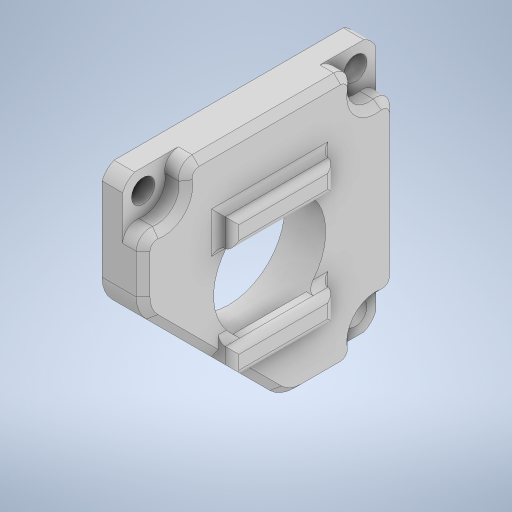
# Autodesk Inventor part: X-Axis-Motor-Support v0.1
Saved by Autodesk Inventor 2023 (Build 270158000, 158)
## iProperties
Created: 2023-07-26
Part Number: X-Axis-Motor-Support v0.1
Material: Generic
Document SubType Name: Modeling
Designer: Parker
Density: 1 g/cm^3
Appearance: Default
Author: Parker
Autodesk Inventor part; units mm, degrees
ref_plane "YZ Plane" through (0, 0, 0) normal (1, 0, 0) x (0, 1, 0)
ref_plane "XZ Plane" through (0, 0, 0) normal (0, 1, 0) x (-1, 0, 0)
ref_plane "XY Plane" through (0, 0, 0) normal (0, 0, 1) x (1, 0, 0)
sketch "Sketch1" plane through (0, 0, 0) normal (1, 0, 0) x (0, 1, 0)
  circle A0 centre (0, 0) radius 8 construction
  circle A1 centre (0, 0) radius 8.2
  line L0 (-15.5, 15.5) -> (15.5, 15.5) construction
  line L1 (15.5, 15.5) -> (15.5, -15.5) construction
  line L2 (15.5, -15.5) -> (-15.5, -15.5) construction
  line L3 (-15.5, -15.5) -> (-15.5, 15.5) construction
  line L4 (-15.5, 15.5) -> (15.5, -15.5) construction
  line L5 (15.5, 15.5) -> (-15.5, -15.5) construction
  line L6 (-18.5, 18.5) -> (18.5, 18.5)
  line L7 (18.5, 18.5) -> (18.5, -18.5)
  line L8 (18.5, -18.5) -> (-18.5, -18.5)
  line L9 (-18.5, -18.5) -> (-18.5, 18.5)
  line L10 (-18.5, 18.5) -> (18.5, -18.5) construction
  line L11 (18.5, 18.5) -> (-18.5, -18.5) construction
  line L12 (-18.5, -2.5) -> (2.5, 18.5)
  point P0 (-15.5, -15.5)
  dimension "d0" = 16
  dimension "d1" = 0.2
  dimension "d2" = 31
  dimension "d3" = 31
  dimension "d4" = 3
  dimension "d5" = 3
  dimension "d6" = 16
  constraints: 26 end point, 5 coincident, 5 parallel, 4 midpoint, 2 centre point, 2 horizontal, 2 perpendicular, 2 point on line
  measures "d0" diameter of A0
  measures "d1" radial gap between concentric circles of A0 A1
  measures "d2" distance of L0.end L1.end
  measures "d3" distance of L0.start L0.end
  measures "d4" distance from line of L8 L1.end
  measures "d5" distance between parallel lines of L7 L1
  measures "d6" distance of L6.end L12.end
extrude "Extrusion1" add sketch "Sketch1" along normal blind 6 contours L6 L7 L8 L9 L12
sketch "Sketch2" plane through (6, 0, 0) normal (1, 0, 0) x (0, 0, -1)
  point P0 (0, 0)
  point P1 (-15.5, 15.5)
  point P2 (15.5, 15.5)
  point P3 (15.5, -15.5)
hole "Hole1" at (6, 15.5, 15.5) at (6, 15.5, -15.5) at (6, -15.5, -15.5) direction (-1, 0, 0) diameter 3.4 end through all counterbore diameter 6.5 counterbore depth 3 clearance for "Socket Head Cap Screw" size "M3" standard "Ansi Metric M Profile"
sketch "Sketch3" plane through (6, 0, 0) normal (1, 0, 0) x (0, 0, -1)
  arc A0 (-16.75, 18.5) -> (-18.5, 16.75) centre (-15.5, 15.5) ccw projected
  line L0 (-16.75, 18.5) -> (-18.5, 18.5) projected
  line L1 (-18.5, 18.5) -> (-18.5, 16.75) projected
  arc A1 (18.5, 16.75) -> (16.75, 18.5) centre (15.5, 15.5) ccw projected
  line L2 (18.5, 16.75) -> (18.5, 18.5) projected
  line L3 (18.5, 18.5) -> (16.75, 18.5) projected
  arc A2 (16.75, -18.5) -> (18.5, -16.75) centre (15.5, -15.5) ccw projected
  line L4 (16.75, -18.5) -> (18.5, -18.5) projected
  line L5 (18.5, -18.5) -> (18.5, -16.75) projected
  point P0 (0, 0)
extrude "Extrusion2" cut sketch "Sketch3" against normal through all
fillet "Fillet1" radius 2 6 edges at (4.5, 14.25, 18.5) (4.5, 18.5, 14.25) (4.5, 18.5, -14.25) (4.5, 14.25, -18.5) (4.5, -14.25, -18.5) (4.5, -18.5, -14.25)
fillet "Fillet2" radius 5 2 edges at (3, 2.5, 18.5) (3, -18.5, -2.5)
sketch "Sketch4" plane through (6, 0, 0) normal (1, 0, 0) x (0, 0, -1)
  circle A0 centre (0, 0) radius 8.2 projected
  arc A1 (1.0355, -17.0355) -> (4.5711, -18.5) centre (4.5711, -13.5) ccw projected
  line L0 (4.5711, -18.5) -> (10.3461, -18.5) projected
  arc A2 (10.3461, -18.5) -> (12.3095, -16.119) centre (10.3461, -16.5) ccw projected
  arc A3 (16.119, -12.3095) -> (12.3095, -16.119) centre (15.5, -15.5) ccw projected
  arc A4 (16.119, -12.3095) -> (18.5, -10.3461) centre (16.5, -10.3461) ccw projected
  line L1 (18.5, -10.3461) -> (18.5, 10.3461) projected
  arc A5 (18.5, 10.3461) -> (16.119, 12.3095) centre (16.5, 10.3461) ccw projected
  arc A6 (12.3095, 16.119) -> (16.119, 12.3095) centre (15.5, 15.5) ccw projected
  arc A7 (12.3095, 16.119) -> (10.3461, 18.5) centre (10.3461, 16.5) ccw projected
  line L2 (10.3461, 18.5) -> (-10.3461, 18.5) projected
  arc A8 (-10.3461, 18.5) -> (-12.3095, 16.119) centre (-10.3461, 16.5) ccw projected
  arc A9 (-16.119, 12.3095) -> (-12.3095, 16.119) centre (-15.5, 15.5) ccw projected
  arc A10 (-16.119, 12.3095) -> (-18.5, 10.3461) centre (-16.5, 10.3461) ccw projected
  line L3 (-18.5, 10.3461) -> (-18.5, 4.5711) projected
  arc A11 (-18.5, 4.5711) -> (-17.0355, 1.0355) centre (-13.5, 4.5711) ccw projected
  line L4 (-17.0355, 1.0355) -> (1.0355, -17.0355) projected
  line L5 (-7.5, 10.2) -> (7.5, 10.2)
  line L6 (7.5, 10.2) -> (7.5, 6.2)
  line L7 (7.5, 6.2) -> (-7.5, 6.2)
  line L8 (-7.5, 6.2) -> (-7.5, 10.2)
  circle A12 centre (0, 0) radius 8.2 projected
  line L9 (-7.5, 10.2) -> (7.5, 6.2) construction
  line L10 (7.5, 10.2) -> (-7.5, 6.2) construction
  line L11 (-7.5, -6.2) -> (7.5, -6.2)
  line L12 (7.5, -6.2) -> (7.5, -10.2)
  line L13 (7.5, -10.2) -> (-7.5, -10.2)
  line L14 (-7.5, -10.2) -> (-7.5, -6.2)
  line L15 (-7.5, -6.2) -> (7.5, -10.2) construction
  line L16 (7.5, -6.2) -> (-7.5, -10.2) construction
  point P0 (0, 8.2)
  point P1 (0, -8.2)
  point P2 (-7.5, -8.5)
  point P3 (-5.8, -10.2)
  dimension "d20" = 15
  dimension "d21" = 4
  dimension "d22" = 15
  dimension "d23" = 4
  constraints: 24 end point, 4 midpoint, 4 parallel, 2 horizontal, 2 perpendicular, 2 point on circle
  measures "d20" distance of L6.end L7.end
  measures "d21" distance of L5.end L6.end
  measures "d22" distance of L12.end L13.end
  measures "d23" distance of L11.end L12.end
extrude "Extrusion3" add sketch "Sketch4" along normal blind 2 contours L7 A0 | A0 L7 L8 L5 L6 | L11 L12 L13 L4 L14 A0 | A0 L11
chamfer "Chamfer1" distance 1 angle 45 17 edges at (6, 7.4586, 18.5) (6, 2.6577, 18.1194) (6, -3.7322, 12.2678) (6, 11.8892, 17.7724) (6, 13.2019, 13.2019) (6, 17.7724, 11.8892) (6, 18.5, 0) (6, 17.7724, -11.8892) (6, 13.2019, -13.2019) (6, 11.8892, -17.7724) (6, 0, -18.5) (6, -11.8892, -17.7724) (6, -13.2019, -13.2019) (6, -17.7724, -11.8892) (6, -18.5, -7.4586) (6, -18.1194, -2.6577) (6, -13.6178, 2.3822)
fillet "Fillet4" radius 1 17 edges at (8, -7.35, 7.5) (8, -10.2, -0.85) (6, -10.2, -1.5571) (6, -8.2, -7.5) (6, -6.2, -6.4333) (6, -6.2, 6.4333) (8, -6.2, 0) (8, -8.2, -7.5) (6, 10.2, 0) (8, 10.2, 0) (6, 8.2, 7.5) (8, 8.2, 7.5) (6, 6.2, 6.4333) (8, 6.2, 0) (6, 8.2, -7.5) (6, 6.2, -6.4333) (8, 8.2, -7.5)
body "Solid1"
